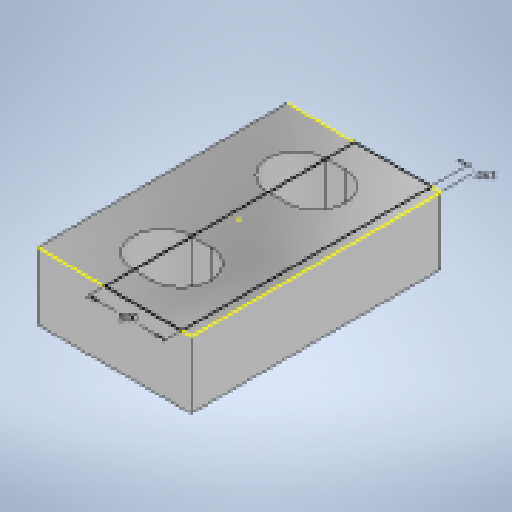
# Autodesk Inventor part: Jaw
Saved by Autodesk Inventor 2023.2 (Build 272271000, 271)
## iProperties
Created: 2024-03-01
Part Number: Jaw
Material: Aluminum 6061
Document SubType Name: Modeling
Designer: Nathan Cai
Density: 2.7 g/cm^3
Appearance: Aluminum - Flat
Author: Nathan Cai
Autodesk Inventor part; units mm, degrees
ref_plane "YZ Plane" through (0, 0, 0) normal (1, 0, 0) x (0, 1, 0)
ref_plane "XZ Plane" through (0, 0, 0) normal (0, 1, 0) x (-1, 0, 0)
ref_plane "XY Plane" through (0, 0, 0) normal (0, 0, 1) x (1, 0, 0)
sketch "Sketch1" plane through (0, 0, 0) normal (0, 1, 0) x (-1, 0, 0)
  line L0 (-15.875, 20.6375) -> (15.875, 20.6375)
  line L1 (15.875, 20.6375) -> (15.875, -20.6375)
  line L2 (15.875, -20.6375) -> (-15.875, -20.6375)
  line L3 (-15.875, -20.6375) -> (-15.875, 20.6375)
  line L4 (-15.875, 20.6375) -> (15.875, -20.6375) construction
  line L5 (15.875, 20.6375) -> (-15.875, -20.6375) construction
  line L6 (0, 20.6375) -> (0, -20.6375) construction
  line L7 (-0.7937, -11.1125) -> (0.7938, -11.1125) construction
  line L8 (-0.7938, -13.6652) -> (0.7937, -13.6652)
  line L9 (0.7938, -8.5598) -> (-0.7937, -8.5598)
  arc A0 (-0.7937, -8.5598) -> (-0.7938, -13.6652) centre (-0.7937, -11.1125) ccw
  arc A1 (0.7937, -13.6652) -> (0.7938, -8.5598) centre (0.7938, -11.1125) ccw
  line L10 (15.875, 0) -> (-15.875, 0) construction
  line L11 (-0.7938, 11.1125) -> (0.7938, 11.1125) construction
  line L12 (-0.7938, 13.6652) -> (0.7937, 13.6652)
  line L13 (0.7938, 8.5598) -> (-0.7937, 8.5598)
  arc A2 (-0.7938, 13.6652) -> (-0.7937, 8.5598) centre (-0.7938, 11.1125) ccw
  arc A3 (0.7938, 8.5598) -> (0.7937, 13.6652) centre (0.7938, 11.1125) ccw
  point P0 (0, 0)
  point P1 (0, -11.1125)
  point P2 (0, 0)
  point P3 (0, 11.1125)
  dimension "d0" = 31.75
  dimension "d1" = 41.275
  dimension "d2" = 0.7937
  dimension "d3" = 5.1054
  dimension "d4" = 11.1125
  constraints: 32 end point, 8 midpoint, 8 point on circle, 7 symmetric about line, 4 centre point, 4 tangent, 3 parallel, 2 perpendicular, 1 horizontal, 1 point on line, 2 other
  measures "d0" distance of L1.end L2.end
  measures "d1" distance of L0.end L1.end
  measures "d2" distance of point (0, -11.113) L7.end
  measures "d3" diameter of A1
  measures "d4" distance from line of point (0, 0) L7
extrude "Extrusion1" add sketch "Sketch1" along normal blind 7.9375
sketch "Sketch2" plane through (0, 7.9375, 0) normal (0, 1, 0) x (1, 0, 0)
  line L0 (15.875, 20.6375) -> (-15.875, 20.6375) projected
  line L1 (-15.875, -20.6375) -> (15.875, -20.6375) projected
  line L2 (14.2875, 20.6375) -> (1.5875, 20.6375)
  line L3 (1.5875, 20.6375) -> (1.5875, -20.6375)
  line L4 (1.5875, -20.6375) -> (14.2875, -20.6375)
  line L5 (14.2875, -20.6375) -> (14.2875, 20.6375)
  line L6 (15.875, -20.6375) -> (15.875, 20.6375) projected
  point P0 (0, 0)
  point P1 (14.2875, -20.6375)
  dimension "d7" = 12.7
  dimension "d8" = 1.5875
  constraints: 8 end point, 2 parallel, 2 point on line, 1 horizontal, 1 perpendicular
  measures "d7" distance of L4.end L3.end
  measures "d8" distance between parallel lines of L6 L5
extrude "Extrusion3" cut sketch "Sketch2" against normal blind 1.5875 contours L6 L1 L5 L0
chamfer "Chamfer1" distance 4.7625 angle 49 8 edges at (0, 7.9375, -13.6652) (3.3464, 7.9375, -11.1125) (0, 7.9375, -8.5598) (-3.3465, 7.9375, -11.1125) (0, 7.9375, 8.5598) (3.3465, 7.9375, 11.1125) (0, 7.9375, 13.6652) (-3.3465, 7.9375, 11.1125) measured on face at (-3.8465, 7.9375, -11.1125) measured on face at (-3.8465, 7.9375, 11.1125) measured on face at (3.8464, 7.9375, -11.1125) measured on face at (0, 7.9375, -8.0598) measured on face at (3.8465, 7.9375, 11.1125) measured on face at (0, 7.9375, -14.1652) measured on face at (0, 7.9375, 14.1652) measured on face at (0, 7.9375, 8.0598)
body "Solid1"
